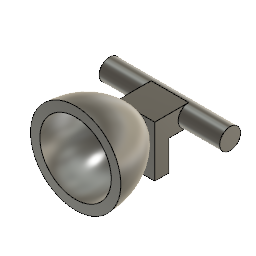
Arm (Autodesk Fusion 360 design; units mm, degrees)
Autodesk Fusion 360 part; units mm, degrees
note: some values were not read from the file. Chosen so that the rebuilt part matches the saved one: where a step ends. Set by a fixed rule: which sketch regions a step uses.
sketch "ForearmPart1" plane through (0, 0, 0) normal (0, 1, 0) x (1, 0, 0)
  ellipse E0 centre (0, 0) end of major axis (70, 0) minor radius 50
  line L0 (-70, 0) -> (70, 0)
  line L1 (0, -50) -> (0, 50)
  line L2 (1.75, 0) -> (22.5, 0)
  ellipse E1 centre (0, 0) end of major axis (80, 0) minor radius 60
  line L3 (-80, 0) -> (80, 0)
  line L4 (0, -60) -> (0, 60)
  dimension "d5" = 140
  dimension "d6" = 50
  dimension "d7" = 10
  dimension "d8" = 10
  constraint coincident E0.centre E1.centre
  constraint coincident E0 L0.start
  constraint coincident E0 L0.end
  constraint coincident E0 L1.start
  constraint coincident E0 L1.end
  constraint parallel L0 L2
  constraint parallel L0 L3
  constraint coincident E1 L3.start
  constraint coincident E1 L3.end
  constraint coincident E1 L4.start
  constraint coincident E1 L4.end
  measures "d5" distance of E0
  measures "d6" distance of L0 L1.start
  measures "d7" distance of L0.end L3.end
  measures "d8" distance of L1.start L4.start
sketch "ForearmReference2" plane through (0, 0, 0) normal (1, 0, 0) x (0, 1, 0)
  line L0 (0, -60) -> (0, 60)
  line L1 (0, 0) -> (-50, 0) construction
  dimension "d9" = 50
  constraint coincident L1.start origin
  constraint perpendicular L0 L1
  measures "d9" distance of L1.start L1.end
extrude "Extrude1" add sketch "ForearmPart1" against normal blind 50 contours E0 E1 L3 L4 | E0 E1 L3 L4 | E0 E1 L3 L4 | E0 E1 L3 L4 makes body 1
sketch "FarearmReferenceHoles" plane through (0, 0, 0) normal (1, 0, 0) x (0, 1, 0)
  circle A0 centre (-25, 0) radius 15
  line L0 (0, 0) -> (-50, 0) construction
  dimension "d12" = 30
  constraint midpoint A0.centre L0
  measures "d12" diameter of A0
extrude "Extrude2" cut sketch "FarearmReferenceHoles" along normal through all and the other way through all bodies 1
sketch "JointHoles" plane through (0, 0, 0) normal (1, 0, 0) x (0, 1, 0)
  circle A0 centre (-25, 0) radius 14
  line L0 (0, 0) -> (-50, 0)
  dimension "d14" = 28
  constraint midpoint A0.centre L0
  measures "d14" diameter of A0
extrude "Extrude3" add sketch "JointHoles" along normal mid plane 160 separate body makes body 2
sketch "Part1ref" plane through (0, -50, 0) normal (0, -1, 0) x (1, 0, 0)
  ellipse E0 centre (0, 0) end of major axis (70, 0) minor radius 50
  ellipse E1 centre (0, 0) end of major axis (80, 0) minor radius 60
  line L0 (-80, 14) -> (-80, -14)
  line L1 (80, -14) -> (80, 14)
  line L2 (-80, 14) -> (80, 14)
  line L3 (-80, -14) -> (80, -14)
  line L4 (-25, 14) -> (25, 14)
  line L5 (25, 14) -> (25, -14)
  line L6 (25, -14) -> (-25, -14)
  line L7 (-25, -14) -> (-25, 14)
  line L8 (-25, 14) -> (25, -14) construction
  line L9 (25, 14) -> (-25, -14) construction
  dimension "d17" = 50
  constraint coincident L0.start L2.start
  constraint coincident L1.end L2.end
  constraint coincident L0.end L3.start
  constraint coincident L1.start L3.end
  constraint horizontal L4
  constraint perpendicular L4 L5
  constraint parallel L4 L6
  constraint parallel L5 L7
  constraint coincident L8 E0.centre
  constraint coincident L9 E0.centre
  constraint coincident E0.centre E1.centre
  constraint collinear L2 L4
  measures "d17" distance of L5.end L6.end
extrude "Extrude4" add sketch "Part1ref" along normal blind 20 and the other way up to far side of body 2 contours L2 L3 L4 L5 L6 L7 bodies 2
sketch "StopperPart1" plane through (0, 0, -14) normal (0, 0, -1) x (1, 0, 0)
  line L0 (25, 25) -> (25, 70)
  line L1 (25, 70) -> (-25, 70)
  line L2 (-25, 70) -> (-25, 25)
  line L3 (-25, 25) -> (25, 25)
  spline S0 degree 3 poles (77.5562, 22.099) (77.5562, 22.099) (77.6208, 21.1271) (77.7181, 20.1629) (78.0822, 17.3945) (78.423, 15.7174) (79.0571, 13.0697) (79.3932, 11.9176) (79.7492, 10.7661) (79.8437, 10.4747) (79.9692, 10.0916) (80, 10) (80, 10) (79.9692, 10.0916) (79.8437, 10.4747) (79.7492, 10.7661) (79.3932, 11.9176) (79.0571, 13.0697) (78.423, 15.7174) (78.0822, 17.3945) (77.7181, 20.1629) (77.6208, 21.1271) (77.4916, 23.0709) (77.4597, 24.0505) (77.4597, 25) knots 0 0.284861 0.284861 0.284861 0.284861 0.569723 0.569723 1.139446 1.139446 1.709028 1.709028 1.993819 1.993819 2.278609 2.278609 2.5634 2.5634 2.848191 2.848191 3.417773 3.417773 3.987496 3.987496 4.272357 4.272357 4.557219 4.557219 4.557219 4.557219
  spline S1 degree 3 poles (-77.5562, 22.099) (-77.5562, 22.099) (-77.6208, 21.1271) (-77.7181, 20.1629) (-78.0822, 17.3945) (-78.423, 15.7174) (-79.0571, 13.0697) (-79.3932, 11.9176) (-79.7492, 10.7661) (-79.8437, 10.4747) (-79.9692, 10.0916) (-80, 10) (-80, 10) (-79.9692, 10.0916) (-79.8437, 10.4747) (-79.7492, 10.7661) (-79.3932, 11.9176) (-79.0571, 13.0697) (-78.423, 15.7174) (-78.0822, 17.3945) (-77.7181, 20.1629) (-77.6208, 21.1271) (-77.4916, 23.0709) (-77.4597, 24.0505) (-77.4597, 25) knots 4.557219 4.84208 4.84208 4.84208 4.84208 5.126942 5.126942 5.696665 5.696665 6.266247 6.266247 6.551037 6.551037 6.835828 6.835828 7.120619 7.120619 7.40541 7.40541 7.974992 7.974992 8.544715 8.544715 8.829576 8.829576 9.114438 9.114438 9.114438 9.114438
  line L4 (80, 50) -> (-80, 50)
  line L5 (-80, 0) -> (80, 0)
  line L6 (25, 70) -> (-25, 70)
  line L7 (-25, 70) -> (-25, 51)
  line L8 (-25, 51) -> (25, 51)
  line L9 (25, 51) -> (25, 70)
  dimension "d24" = 1
  constraint perpendicular L6 L7
  constraint parallel L6 L8
  constraint parallel L7 L9
  constraint coincident L1.end L2.start
  constraint perpendicular L2 L6
  constraint coincident L0.end L1.start
  measures "d24" distance of L4 L8
extrude "Extrude5" add sketch "StopperPart1" along normal blind 40 contours L0 L1 L2 L6 L7 L8 L9 bodies 2
sketch "Stopper" plane through (0, -70, 0) normal (0, -1, 0) x (1, 0, 0)
  line L0 (25, -54) -> (25, 14)
  line L1 (25, 14) -> (-25, 14)
  line L2 (-25, 14) -> (-25, -54)
  line L3 (-25, -54) -> (25, -54)
sketch "Arm Mould" plane through (0, 0, 0) normal (1, 0, 0) x (0, 1, 0)
  line L0 (-50, -50) -> (-50, 50)
  line L1 (-50, 60) -> (-50, -60)
  line L2 (-70, -54) -> (-70, 14)
  line L3 (-70, 14) -> (-70, -54)
  line L4 (-50, 60) -> (-150, 60) construction
  line L5 (-150, 60) -> (-150, 47.3246)
  arc A0 (-70, 14) -> (-150, 60) centre (-150, -32.5652) ccw
  arc A1 (-70, 4) -> (-150, 47.3246) centre (-144.1753, -37.4432) ccw
  dimension "d44" = 100
  dimension "d45" = 10
  dimension "d46" = 84.9677
  constraint horizontal L4
  constraint coincident L1.start L4.start
  constraint perpendicular L4 L5
  constraint tangent L4 A0
  constraint coincident L2.end L3.start
  constraint tangent A0 A1
  constraint coincident L2 A1.start
  measures "d44" distance of L1.start L4.end
  measures "d45" distance of L2.end A1.start
  measures "d46" radius of A1
revolve "Revolve2" add sketch "Arm Mould" angle 360 about axis through (0, 1.75, 0) along (0, 1, 0) bodies 2
hidden bodies 1
equation "d10 = -d9"
equation "d26 = 30 mm"
equation "d27 = 60.00 mm"
equation "d29 = d26 * 1.5"
equation "d30 = d27 * 1.5"
named bodies: "Shell", "Joint"
